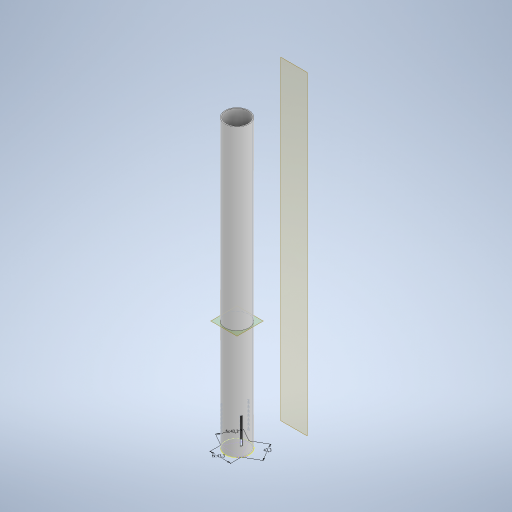
# Autodesk Inventor part: Part1
Saved by Autodesk Inventor 2023.2 (Build 272271000, 271)
## iProperties
Created: 2022-12-18
Part Number: Part1
Material: Generic
Document SubType Name: Modeling
Designer: Admin
Density: 1 g/cm^3
Appearance: Default
Author: Admin
Autodesk Inventor part; units mm, degrees
ref_plane "YZ Plane" through (0, 0, 0) normal (1, 0, 0) x (0, 1, 0)
ref_plane "XZ Plane" through (0, 0, 0) normal (0, 1, 0) x (-1, 0, 0)
sketch "Sketch2" plane through (0, 0, 0) normal (0, 1, 0) x (-1, 0, 0)
  circle A0 centre (0, 0) radius 25
  circle A1 centre (0, 0) radius 23
  dimension "d0" = 50
  dimension "d1" = 46
  constraints: 2 centre point, 2 coincident
  measures "d0" diameter of A0
  measures "d1" diameter of A1
extrude "Extrusion1" add sketch "Sketch2" along normal blind 600
ref_plane "Work Plane1" through (0, 0, -25) normal (0, 0, 1) x (1, 0, 0)
sketch "Sketch3" plane through (0, 0, -25) normal (0, 0, 1) x (1, 0, 0)
  line L0 (-25, 0) -> (-25, 600) projected
  line L1 (25, 0) -> (-25, 0) projected
  line L2 (1.6, 20) -> (-1.6, 20)
  line L3 (-1.6, 20) -> (-1.6, 75)
  line L4 (-1.6, 75) -> (1.6, 75)
  line L5 (1.6, 75) -> (1.6, 20)
  point P0 (0, 0)
  point P1 (0, 75)
  dimension "d4" = 600
  dimension "d5" = 50
  dimension "d6" = 3.2
  dimension "d7" = 55
  dimension "d8" = 20
  dimension "d9" = 25
  constraints: 8 end point, 2 parallel, 1 horizontal, 1 midpoint, 1 perpendicular
  measures "d4" distance of L0.start L0.end
  measures "d5" distance of L1.start L0.start
  measures "d6" distance of L3.end L4.end
  measures "d7" distance of L2.end L3.end
  measures "d8" distance from line of L1 L2.end
  measures "d9" distance from line of L0 point (0, 75)
extrude "Extrusion2" cut sketch "Sketch3" along normal mid plane 10
sketch "Sketch4" plane through (0, 0, 0) normal (0, 1, 0) x (-1, 0, 0)
  circle A0 centre (0, 0) radius 25 projected
  line L0 (0, -25) -> (-21.65, 12.4989) construction
  line L1 (-21.65, 12.4989) -> (21.65, 12.4989) construction
  line L2 (21.65, 12.4989) -> (0, -25) construction
  line L3 (-17.6606, 19.4109) -> (-26.5815, 3.9594) construction
  line L4 (20.7261, 14.1013) -> (22.5717, 10.9047) construction
  dimension "d12" = 43.3
  dimension "d13" = 43.3
  dimension "d14" = 43.3
  constraints: 10 end point, 1 horizontal, 1 vertical alignment, 3 other
  measures "d12" distance of L1.end L0.start
  measures "d13" distance of L0.start L0.end
  measures "d14" distance of L0.end L1.end
pattern_circular "Circular Pattern1" count 3 over 360 about axis through (0, 0, 0) along (0, 1, 0) of "Extrusion2"
ref_plane "Work Plane14" through (0, 230, 0) normal (0, -1, 0) x (1, 0, 0)
split_face "Split6"
equation "\"d12\" = d14"
equation "\"d14\" = d13"
body "Solid1"
